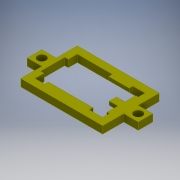
# Autodesk Inventor part: TP4056_long_holder
Saved by Autodesk Inventor 2018 (Build 220112000, 112)
## iProperties
Created: 2019-09-05
Part Number: TP4056_long_holder
Material: Generic
Document SubType Name: Modeling
Designer: ZEUSLAP
Density: 1 g/cm^3
Appearance: Default
Author: ZEUSLAP
## iProperties of the stored document TP4056_long_holder_3DPrint.ipt
Created: 2019-09-05
Part Number: TP4056_long_holder_3DPrint
Material: Generic
Document SubType Name: Modeling
Designer: ZEUSLAP
Density: 1 g/cm^3
Appearance: Default
Author: ZEUSLAP
Autodesk Inventor part; units mm, degrees
ref_plane "YZ Plane" through (0, 0, 0) normal (1, 0, 0) x (0, 1, 0)
ref_plane "XZ Plane" through (0, 0, 0) normal (0, 1, 0) x (-1, 0, 0)
ref_plane "XY Plane" through (0, 0, 0) normal (0, 0, 1) x (1, 0, 0)
sketch "shape" plane through (0, 0, 0) normal (0, 0, 1) x (1, 0, 0)
  line L0 (-14, 8.75) -> (14, 8.75)
  line L1 (14, 8.75) -> (14, -8.75)
  line L2 (14, -8.75) -> (-14, -8.75)
  line L3 (-14, -8.75) -> (-14, 8.75)
  line L4 (17, 11.75) -> (-17, 11.75)
  line L5 (-17, 11.75) -> (-17, -11.75)
  line L6 (-17, -11.75) -> (17, -11.75)
  line L7 (17, -11.75) -> (17, 11.75)
  line L8 (-15.5, 5) -> (-14, 5)
  line L9 (-14, 5) -> (-14, -5)
  line L10 (-14, -5) -> (-15.5, -5)
  line L11 (-15.5, -5) -> (-15.5, 5)
  line L12 (-10, -7.25) -> (8.5, -7.25)
  line L13 (8.5, -7.25) -> (8.5, -8.75)
  line L14 (8.5, -8.75) -> (-10, -8.75)
  line L15 (-10, -8.75) -> (-10, -7.25)
  line L16 (13, 6) -> (14, 6)
  line L17 (14, 6) -> (14, -6)
  line L18 (14, -6) -> (13, -6)
  line L19 (13, -6) -> (13, 6)
  line L20 (9.5, 1.5) -> (13, 1.5)
  line L21 (13, 1.5) -> (13, -1.5)
  line L22 (13, -1.5) -> (9.5, -1.5)
  line L23 (9.5, -1.5) -> (9.5, 1.5)
  line L24 (0.5, 8.75) -> (9, 8.75)
  line L25 (9, 8.75) -> (9, 7.25)
  line L26 (9, 7.25) -> (0.5, 7.25)
  line L27 (0.5, 7.25) -> (0.5, 8.75)
  line L28 (-23, 3) -> (-17, 3)
  line L29 (-17, 3) -> (-17, -3)
  line L30 (-17, -3) -> (-23, -3)
  line L31 (-23, -3) -> (-23, 3)
  line L32 (17, 3) -> (23, 3)
  line L33 (23, 3) -> (23, -3)
  line L34 (23, -3) -> (17, -3)
  line L35 (17, -3) -> (17, 3)
  circle A0 centre (-20, 0) radius 1.75
  circle A1 centre (20, 0) radius 1.75
  point P0 (0, 0)
  point P1 (0, 8.75)
  point P2 (14, 0)
  point P3 (-15.5, 0)
  point P4 (13, 0)
  point P5 (9.5, 0)
  point P6 (-17, 0)
  point P7 (17, 0)
  point P8 (-17, 0)
  point P9 (17, 0)
  point P10 (20, 3)
  point P11 (-20, 3)
  dimension "d0" = 28
  dimension "d1" = 17.5
  dimension "d2" = 3
  dimension "d3" = 1.5
  dimension "d4" = 10
  dimension "d5" = 18.5
  dimension "d6" = 1.5
  dimension "d7" = 4
  dimension "d8" = 1
  dimension "d9" = 12
  dimension "d10" = 3.5
  dimension "d11" = 3
  dimension "d12" = 8.5
  dimension "d13" = 1.5
  dimension "d14" = 5
  dimension "d19" = 6
  dimension "d22" = 3.5
  constraints: 72 end point, 18 parallel, 11 midpoint, 9 perpendicular, 8 horizontal, 8 horizontal alignment, 7 collinear, 3 equal length, 3 vertical alignment, 2 centre point, 1 equal radius, 3 other
  measures "d0" distance of L1.end L2.end
  measures "d1" distance of L0.end L1.end
  measures "d2" distance between parallel lines of L0 L4
  measures "d3" distance of L9.end L10.end
  measures "d4" distance of L8.end L9.end
  measures "d5" distance of L13.end L14.end
  measures "d6" distance of L12.end L13.end
  measures "d7" distance between parallel lines of L3 L15
  measures "d8" distance of L17.end L18.end
  measures "d9" distance of L16.end L17.end
  measures "d10" distance of L21.end L22.end
  measures "d11" distance of L20.end L21.end
  measures "d12" distance of L25.end L26.end
  measures "d13" distance of L24.end L25.end
  measures "d14" distance between parallel lines of L1 L25
  measures "d19" distance of L29.end L30.end
  measures "d22" diameter of A1
extrude "around pcb" add sketch "shape" against normal blind 1.5 contours L1 L18 L19 L16 | L7 L6 L5 L4 | L32 L33 L34 L7 | L5 L30 L31 L28
extrude "over pcb" add sketch "shape" along normal blind 1.5 contours L0 L25 L26 L27 | L1 L18 L19 L16 | L15 L12 L13 L2 | L19 L22 L23 L20 | L7 L6 L5 L4 | L32 L33 L34 L7 | L5 L30 L31 L28
body "Solid1"
